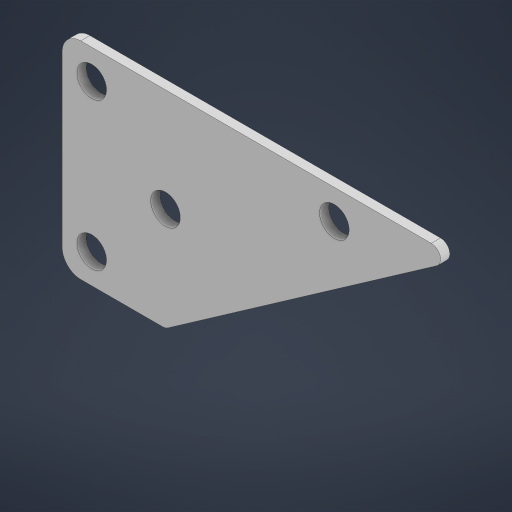
# Autodesk Inventor part: Sleds poly V3
Saved by Autodesk Inventor 2023.4 (Build 274418000, 418)
## iProperties
Created: 2024-01-28
Part Number: Sleds poly V3
Material: Generic
Document SubType Name: Modeling
Designer: diego
Density: 1 g/cm^3
Appearance: Default
Author: diego
Autodesk Inventor part; units mm, degrees
ref_plane "YZ Plane" through (0, 0, 0) normal (1, 0, 0) x (0, 1, 0)
ref_plane "XZ Plane" through (0, 0, 0) normal (0, 1, 0) x (-1, 0, 0)
ref_plane "XY Plane" through (0, 0, 0) normal (0, 0, 1) x (1, 0, 0)
sketch "Sketch1" plane through (0, 0, 0) normal (0, 0, 1) x (1, 0, 0)
  line L0 (-23.2284, 21.8872) -> (-18.1484, 21.8872)
  line L1 (-23.2284, -16.2062) -> (-18.1484, -16.2062)
  circle A0 centre (-18.1484, -16.2062) radius 2.54
  line L2 (-18.1484, 21.8872) -> (19.9486, 21.8872)
  line L3 (-5.4453, 21.8872) -> (-5.4453, 9.1863)
  line L4 (-18.1484, -16.2062) -> (19.9486, -16.2062)
  line L5 (-18.1484, -16.2062) -> (-18.1484, -21.2862)
  line L6 (-18.1484, -16.2062) -> (-18.1484, -3.5079)
  circle A1 centre (-18.1484, -3.5079) radius 2.54
  circle A2 centre (-18.1484, 9.1863) radius 2.54
  line L7 (-18.1484, -3.5079) -> (-18.1484, 9.1863)
  line L8 (-18.1484, 9.1863) -> (-18.1484, 14.2578)
  line L9 (-18.1484, 14.2578) -> (-23.2284, 14.2578)
  line L10 (-18.1484, 9.1863) -> (-23.2284, 9.1863)
  line L11 (-23.2284, 9.1863) -> (-23.2284, 14.2578)
  line L12 (-23.2284, -16.2062) -> (-23.2284, 9.1863)
  line L13 (-18.1484, -21.2862) -> (-23.2284, -21.2862)
  line L14 (-23.2284, -21.2862) -> (-23.2284, -16.2062)
  line L15 (-18.1484, -16.2062) -> (-5.4453, -16.2062)
  line L16 (-5.4453, -16.2062) -> (-5.4453, -3.51)
  line L17 (-5.4453, -3.51) -> (-5.4453, 9.1863)
  circle A3 centre (-5.4453, 9.1863) radius 2.54
  circle A4 centre (-5.4453, -3.51) radius 2.54
  circle A5 centre (-5.4453, -16.2062) radius 2.54
  line L18 (-18.1484, -21.2862) -> (-5.4453, -21.2862)
  line L19 (-5.4453, -21.2862) -> (-5.4453, -16.2062)
  line L20 (-18.1484, 14.2578) -> (51.4388, 14.2578)
  line L21 (-5.4453, 9.1863) -> (32.6494, 9.1863)
  line L22 (51.4388, 14.2578) -> (70.7651, 14.2578)
  line L23 (-5.4453, -21.2862) -> (340.0859, 220.6448)
  circle A6 centre (23.6039, 9.1863) radius 2.54
  point P0 (0, 0)
  point P1 (-18.1484, 11.7263)
  point P2 (-20.6884, 9.1863)
  point P3 (-18.1484, 6.6463)
  point P4 (45.3195, 14.2578)
  dimension "d0" = 5.08
  dimension "d1" = 5.08
  dimension "d3" = 5.08
  dimension "d4" = 5.08
  dimension "d5" = 5.08
  dimension "d6" = 5.08
  dimension "d7" = 5.08
  dimension "d8" = 5.08
  dimension "d19" = 5.08
  constraints: 48 end point, 8 horizontal, 7 centre point, 7 perpendicular, 6 coincident, 5 point on line, 3 vertical, 1 collinear, 1 parallel
  measures "d0" distance of L0.start L0.end
  measures "d1" diameter of A0
  measures "d3" distance of L4.start L5.end
  measures "d4" diameter of A1
  measures "d5" diameter of A2
  measures "d6" diameter of A3
  measures "d7" diameter of A4
  measures "d8" diameter of A5
  measures "d19" diameter of A6
extrude "Extrusion2" add sketch "Sketch1" along normal blind 1.5875 contours L12 L10 A2 L7 A1 L6 A0 L1 | L1 A0 L5 L13 L14 | L11 L9 L8 A2 L10 | L6 A1 L7 A2 L8 L20 L3 A3 L17 A4 L16 A5 L4 A0 | A0 L4 A5 L19 L18 L5 | A1 L7 L6 | L6 L7 A1 | L19 A5 L4 L23 | A5 L16 L4 | L4 L19 A5 | L20 L23 L4 A5 L16 A4 L17 A3 L3 | L19 L4 A5 | L16 A5 L4 | A3 L21 L3 | L3 L17 A3 | L21 A3 L17
fillet "Fillet5" radius 1.5875 2 edges at (45.3195, 14.2578, 0.7937) (-5.4453, -21.2862, 0.7937)
fillet "Fillet6" radius 3.175 2 edges at (-23.2284, 14.2578, 0.7937) (-23.2284, -21.2862, 0.7937)
body "Solid2"
